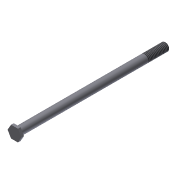
# Autodesk Inventor part: 375 bolt x4
Saved by Autodesk Inventor 2013 (Build 170138000, 138)
## iProperties
Created: 2011-07-05
Part Number: 375 bolt x4
Document SubType Name: Modeling
Designer: Dan Niemitalo
Density: 7.85 g/cm^3
Material: Steel
Mass: 103.831 g
Surface Area: 58.219 cm^2
Volume: 13.2268 cm^3
Author: Dan Niemitalo
Autodesk Inventor part; units mm, degrees
ref_plane "YZ Plane" through (0, 0, 0) normal (1, 0, 0) x (0, 1, 0)
ref_plane "XZ Plane" through (0, 0, 0) normal (0, 1, 0) x (-1, 0, 0)
ref_plane "XY Plane" through (0, 0, 0) normal (0, 0, 1) x (1, 0, 0)
sketch "Sketch1" plane through (0, 0, 0) normal (0, 0, 1) x (1, 0, 0)
  circle A0 centre (-414.4261, -56.251) radius 4.7625
  point P0 (0, 0)
  dimension "d0" = 9.525
  constraints: 1 centre point
  measures "d0" diameter of A0
extrude "Extrusion1" add sketch "Sketch1" against normal blind 177.8
sketch "Sketch2" plane through (-414.4261, -56.251, 0) normal (0, 0, 1) x (1, 0, 0)
  circle A0 centre (0, 0) radius 4.7625 projected
  line L0 (-8.2489, 0) -> (-4.1244, 7.1437)
  line L1 (-4.1244, 7.1437) -> (4.1244, 7.1438)
  line L2 (4.1244, 7.1438) -> (8.2489, 0)
  line L3 (8.2489, 0) -> (4.1244, -7.1437)
  line L4 (4.1244, -7.1437) -> (-4.1244, -7.1438)
  line L5 (-4.1244, -7.1438) -> (-8.2489, 0)
  point P0 (414.4261, 56.251)
  dimension "d3" = 14.2875
  constraints: 12 end point, 1 coincident, 13 other
  measures "d3" distance between parallel lines of L4 L1
extrude "Extrusion2" add sketch "Sketch2" along normal blind 3.175 contours A0 | L0 L1 L2 L3 L4 L5
thread "Thread1" size "3/8-16 UNC" class "2A" standard "ANSI Unified Screw Threads" length 25.4
chamfer "Chamfer1" distance 0.508 angle 45 1 edges at (-419.1886, -56.251, -177.8)
body "Solid1"
